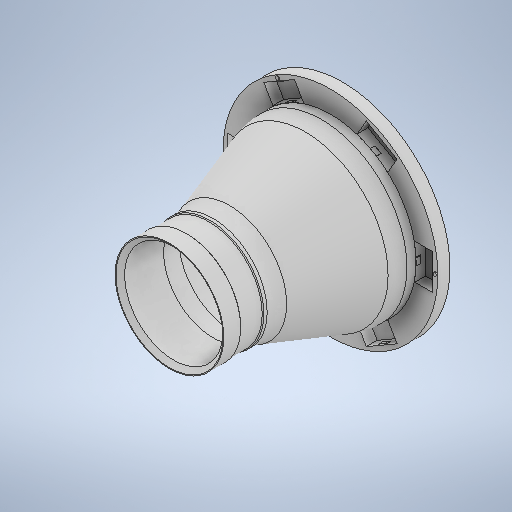
# Autodesk Inventor part: 4-2.5inchConvertor
Saved by Autodesk Inventor 2025.2 (Build 292293000, 293)
## iProperties
Created: 2024-12-23
Part Number: 4-2.5inchConvertor
Material: Generic
Document SubType Name: Modeling
Designer: lidang
Density: 1 g/cm^3
Appearance: Default
Author: lidang
Autodesk Inventor part; units mm, degrees
ref_plane "YZ Plane" through (0, 0, 0) normal (1, 0, 0) x (0, 1, 0)
ref_plane "XZ Plane" through (0, 0, 0) normal (0, 1, 0) x (-1, 0, 0)
sketch "Sketch1" plane through (0, 0, 0) normal (0, 0, 1) x (1, 0, 0)
  circle A0 centre (0, 0) radius 46.465
  line L0 (48.75, 10.25) -> (59.25, 10.25)
  line L1 (59.25, 10.25) -> (59.25, -10.25)
  line L2 (59.25, -10.25) -> (48.75, -10.25)
  line L3 (48.75, -10.25) -> (48.75, 10.25)
  circle A1 centre (0, 0) radius 62
  line L4 (59.25, 2) -> (58.75, 2)
  line L5 (58.75, 2) -> (58.75, -2)
  line L6 (58.75, -2) -> (59.25, -2)
  line L7 (59.25, -2) -> (59.25, 2)
  line L8 (54, 10.25) -> (54, -10.25)
  line L9 (48.75, 2) -> (49.25, 2)
  line L10 (49.25, 2) -> (49.25, -2)
  line L11 (49.25, -2) -> (48.75, -2)
  line L12 (48.75, -2) -> (48.75, 2)
  line L13 (27.8929, 52.312) -> (27.6429, 51.879)
  line L14 (31.1071, 49.879) -> (31.3571, 50.312)
  line L15 (31.3571, 50.312) -> (27.8929, 52.312)
  line L16 (27.6429, 51.879) -> (31.1071, 49.879)
  line L17 (22.6429, 43.2187) -> (22.8929, 43.6518)
  line L18 (22.8929, 43.6518) -> (26.3571, 41.6518)
  line L19 (26.1071, 41.2187) -> (22.6429, 43.2187)
  line L20 (26.3571, 41.6518) -> (26.1071, 41.2187)
  line L21 (33.2518, 37.0937) -> (15.4982, 47.3437)
  line L22 (38.5018, 46.187) -> (33.2518, 37.0937)
  line L23 (20.7482, 56.437) -> (38.5018, 46.187)
  line L24 (15.4982, 47.3437) -> (20.7482, 56.437)
  line L25 (-31.3571, 50.312) -> (-31.1071, 49.879)
  line L26 (-27.6429, 51.879) -> (-27.8929, 52.312)
  line L27 (-27.8929, 52.312) -> (-31.3571, 50.312)
  line L28 (-31.1071, 49.879) -> (-27.6429, 51.879)
  line L29 (-26.1071, 41.2187) -> (-26.3571, 41.6518)
  line L30 (-26.3571, 41.6518) -> (-22.8929, 43.6518)
  line L31 (-22.6429, 43.2187) -> (-26.1071, 41.2187)
  line L32 (-22.8929, 43.6518) -> (-22.6429, 43.2187)
  line L33 (-15.4982, 47.3437) -> (-33.2518, 37.0937)
  line L34 (-20.7482, 56.437) -> (-15.4982, 47.3437)
  line L35 (-38.5018, 46.187) -> (-20.7482, 56.437)
  line L36 (-33.2518, 37.0937) -> (-38.5018, 46.187)
  line L37 (-59.25, -2) -> (-58.75, -2)
  line L38 (-58.75, 2) -> (-59.25, 2)
  line L39 (-59.25, 2) -> (-59.25, -2)
  line L40 (-58.75, -2) -> (-58.75, 2)
  line L41 (-48.75, -2) -> (-49.25, -2)
  line L42 (-49.25, -2) -> (-49.25, 2)
  line L43 (-48.75, 2) -> (-48.75, -2)
  line L44 (-49.25, 2) -> (-48.75, 2)
  line L45 (-48.75, 10.25) -> (-48.75, -10.25)
  line L46 (-59.25, 10.25) -> (-48.75, 10.25)
  line L47 (-59.25, -10.25) -> (-59.25, 10.25)
  line L48 (-48.75, -10.25) -> (-59.25, -10.25)
  line L49 (-27.8929, -52.312) -> (-27.6429, -51.879)
  line L50 (-31.1071, -49.879) -> (-31.3571, -50.312)
  line L51 (-31.3571, -50.312) -> (-27.8929, -52.312)
  line L52 (-27.6429, -51.879) -> (-31.1071, -49.879)
  line L53 (-22.6429, -43.2187) -> (-22.8929, -43.6518)
  line L54 (-22.8929, -43.6518) -> (-26.3571, -41.6518)
  line L55 (-26.1071, -41.2187) -> (-22.6429, -43.2187)
  line L56 (-26.3571, -41.6518) -> (-26.1071, -41.2187)
  line L57 (-33.2518, -37.0937) -> (-15.4982, -47.3437)
  line L58 (-38.5018, -46.187) -> (-33.2518, -37.0937)
  line L59 (-20.7482, -56.437) -> (-38.5018, -46.187)
  line L60 (-15.4982, -47.3437) -> (-20.7482, -56.437)
  line L61 (31.3571, -50.312) -> (31.1071, -49.879)
  line L62 (27.6429, -51.879) -> (27.8929, -52.312)
  line L63 (27.8929, -52.312) -> (31.3571, -50.312)
  line L64 (31.1071, -49.879) -> (27.6429, -51.879)
  line L65 (26.1071, -41.2187) -> (26.3571, -41.6518)
  line L66 (26.3571, -41.6518) -> (22.8929, -43.6518)
  line L67 (22.6429, -43.2187) -> (26.1071, -41.2187)
  line L68 (22.8929, -43.6518) -> (22.6429, -43.2187)
  line L69 (15.4982, -47.3437) -> (33.2518, -37.0937)
  line L70 (20.7482, -56.437) -> (15.4982, -47.3437)
  line L71 (38.5018, -46.187) -> (20.7482, -56.437)
  line L72 (33.2518, -37.0937) -> (38.5018, -46.187)
  circle A2 centre (0, 0) radius 49.465
  point P0 (35.8768, 41.6404)
  point P1 (18.1232, 51.8904)
  point P2 (-18.1232, 51.8904)
  point P3 (-35.8768, 41.6404)
  point P4 (-54, 10.25)
  point P5 (-54, -10.25)
  point P6 (-35.8768, -41.6404)
  point P7 (-18.1232, -51.8904)
  point P8 (18.1232, -51.8904)
  point P9 (35.8768, -41.6404)
  dimension "d1" = 92.93
  dimension "d16" = 20.5
  dimension "d17" = 10.5
  dimension "d71" = 54
  dimension "d72" = 10.25
  dimension "d73" = 124
  dimension "d74" = 4
  dimension "d75" = 0.5
  dimension "d76" = 2
  dimension "d83" = 360
  dimension "d85" = 98.93
  constraints: 146 end point, 6 point on line, 4 parallel, 4 symmetric about line, 3 centre point, 2 horizontal, 2 midpoint, 2 perpendicular, 1 coincident, 157 other
  measures "d1" diameter of A0
  measures "d16" distance of L0.end L1.end
  measures "d17" distance of L1.end L2.end
  measures "d71" horizontal distance of point (0, 0) L8.start
  measures "d72" vertical distance of point (0, 0) L8.start
  measures "d73" diameter of A1
  measures "d74" distance of L4.end L5.end
  measures "d75" distance of L5.end L6.end
  measures "d76" vertical distance of point (0, 0) L5.end
  measures "d85" diameter of A2
extrude "Extrusion9" add sketch "Sketch1" along normal blind 7 contours A0 | L0 L8 L2 L3 A2 | L0 L1 L4 L5 L6 L2 L8 | A2 L3 L11 L10 L9 | L3 A2 L69 L67 L57 L55 L45 L43 L33 L31 L21 L19 | L9 L10 L11 L3 | A2 L21 L24 L23 L13 L16 L14 L22 | L21 L20 L18 L17 A2 | L1 L6 L5 L4 | L19 L17 L18 L20 | A2 L69 L68 L66 L65 | L69 L72 L71 L61 L64 L62 L70 A2 | A2 L33 L36 L35 L25 L28 L26 L34 | L33 L32 L30 L29 A2 | L65 L66 L68 L67 | L14 L16 L13 L15 | L31 L29 L30 L32 | A2 L57 L56 L54 L53 | L57 L60 L59 L49 L52 L50 L58 A2 | A2 L45 L48 L47 L37 L40 L38 L46 | L45 L44 L42 L41 A2 | L63 L62 L64 L61 | L53 L54 L56 L55 | L26 L28 L25 L27 | L43 L41 L42 L44 | L51 L50 L52 L49 | L38 L40 L37 L39 | A1
extrude "Extrusion11" cut sketch "Sketch1" along normal blind 36 contours A0
extrude "Extrusion12" cut sketch "Sketch1" along normal blind 7 contours A2 L45 L48 L47 L37 L40 L38 L46 | L45 L44 L42 L41 A2 | L43 L41 L42 L44 | L38 L40 L37 L39
extrude "Extrusion13" add sketch "Sketch1" along normal blind 7 contours L43 L41 L42 L44 | L38 L40 L37 L39
extrude "Extrusion14" add sketch "Sketch1" along normal blind 0.75 contours A2 L45 L48 L47 L37 L40 L38 L46 | L45 L44 L42 L41 A2 | L43 L41 L42 L44 | L38 L40 L37 L39
chamfer "Chamfer4" distance 0.5 angle 45 1 edges at (-58.75, 0, 7)
pattern_circular "Circular Pattern3" count 6 over 360 about axis through (0, 0, 0) along (0, 0, 1) of "Extrusion12", "Extrusion13", "Extrusion14", "Chamfer4"
sketch "Sketch3" plane through (0, 0, 7) normal (0, 0, 1) x (1, 0, 0)
  circle A0 centre (60.75, 0) radius 1
  line L0 (59.25, -2) -> (59.25, 2) projected
  point P0 (0, 0)
  dimension "d107" = 2
  dimension "d108" = 1.5
  constraints: 1 centre point
  measures "d107" diameter of A0
  measures "d108" distance from line of L0 A0.centre
extrude "Extrusion15" add sketch "Sketch3" along normal blind 0.5
pattern_circular "Circular Pattern4" count 3 over 360 about axis through (0, 0, 0) along (0, 0, 1) of "Extrusion15"
ref_plane "Work Plane1" through (0, 0, 100) normal (0, 0, 1) x (1, 0, 0)
sketch "Sketch6" plane through (0, 0, 0) normal (0, 1, 0) x (-1, 0, 0)
  line L0 (49.465, 7) -> (49.409, 12.208)
  line L1 (47.816, 21.5364) -> (32.9447, 65.3063)
  arc A0 (49.409, 12.208) -> (47.816, 21.5364) centre (19.4107, 11.8855) ccw
  line L2 (31.35, 74.9573) -> (31.35, 76.839)
  arc A1 (31.35, 74.9573) -> (32.9447, 65.3063) centre (61.35, 74.9573) ccw
  line L3 (0, 100) -> (0, 7)
  line L4 (-46.465, 7) -> (46.465, 7) projected
  line L5 (28.35, 100) -> (28.35, 74.9573)
  arc A2 (28.35, 74.9573) -> (30.1042, 64.3412) centre (61.35, 74.9573) ccw
  line L6 (30.1042, 64.3412) -> (44.9755, 20.5713)
  arc A3 (46.4092, 12.1757) -> (44.9755, 20.5713) centre (19.4107, 11.8855) ccw
  line L7 (46.4092, 12.1757) -> (46.4648, 7)
  line L8 (31.35, 100) -> (28.35, 100)
  line L9 (49.465, 7) -> (46.4648, 7)
  line L10 (48.75, 0.75) -> (48.75, 7) projected
  line L11 (30.85, 89.761) -> (30.85, 89.761)
  line L12 (30.85, 89.761) -> (30.85, 77.339)
  line L13 (30.85, 77.339) -> (30.85, 77.339)
  line L14 (31.35, 90.261) -> (31.35, 100)
  line L15 (31.35, 76.839) -> (30.85, 77.339)
  line L16 (31.35, 90.261) -> (30.85, 89.761)
  point P0 (0, 0)
  point P1 (49.3575, 16.9994)
  point P2 (31.35, 89.761)
  point P3 (31.35, 77.339)
  dimension "d118" = 10
  dimension "d119" = 30
  dimension "d120" = 30
  dimension "d121" = 3
  dimension "d123" = 0.5
  dimension "d124" = 0.5
  dimension "d125" = 0.5
  dimension "d126" = 0.5
  constraints: 30 end point, 8 point on circle, 7 point on line, 5 tangent, 4 centre point, 2 horizontal, 2 perpendicular, 2 vertical, 1 midpoint, 1 parallel, 3 other
  measures "d118" distance of L0.start point (49.357, 16.999)
  measures "d119" radius of A0
  measures "d120" radius of A1
  measures "d121" distance between parallel lines of L2 L5
  measures "d123" distance of L2.end point (31.35, 77.339)
  measures "d124" distance of L13.end point (31.35, 77.339)
  measures "d125" distance of L14.start point (31.35, 89.761)
  measures "d126" distance of L11.start point (31.35, 89.761)
revolve "Revolution1" add sketch "Sketch6" angle 360 about axis through (0, 0, 100) along (0, 0, -1)
sketch "Sketch7" plane through (0, 0, 0.75) normal (0, 0, 1) x (1, 0, 0)
  line L0 (-58.75, 2) -> (-59.25, 2) projected
  line L1 (-59.25, 2) -> (-59.25, -2) projected
  line L2 (-59.25, -2) -> (-58.75, -2) projected
  line L3 (-58.75, -2) -> (-58.75, 2) projected
  line L4 (-48.75, 10.25) -> (-48.75, 2) projected
  line L5 (-49.25, -2) -> (-48.75, -2) projected
  line L6 (-48.75, 2) -> (-49.25, 2)
  line L7 (-49.25, 2) -> (-49.25, -2)
  line L8 (-49.25, -2) -> (-48.75, -2)
  line L9 (-48.75, -2) -> (-48.75, 2)
  point P0 (0, 0)
  point P1 (-49.25, 2)
  constraints: 8 end point, 2 parallel, 1 horizontal, 1 perpendicular
extrude "Extrusion16" cut sketch "Sketch7" along normal blind 3
pattern_circular "Circular Pattern5" count 6 over 360 about axis through (0, 0, 0) along (0, 0, 1) of "Extrusion16"
chamfer "Chamfer6" distance 0.5 angle 45 12 edges at (-58.75, 0, 3.75) (-49.25, 0, 3.75) (-24.625, -42.6518, 3.75) (-29.375, -50.879, 3.75) (24.625, -42.6518, 3.75) (29.375, -50.879, 3.75) (49.25, 0, 3.75) (58.75, 0, 3.75) (24.625, 42.6518, 3.75) (29.375, 50.879, 3.75) (-24.625, 42.6518, 3.75) (-29.375, 50.879, 3.75)
chamfer "Chamfer7" distance 2.5 angle 45 1 edges at (28.35, 0, 100)
equation "\"d72\" = 0.5 * d16"
equation "\"d76\" = 0.5 * d74"
equation "\"d124\" = d123"
equation "\"d125\" = d123"
equation "\"d126\" = d125"
body "Solid2"
